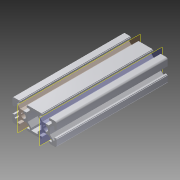
# Autodesk Inventor part: Dual Slotted Extrusion
Saved by Autodesk Inventor 2015 SP1 (Build 190203100, 203)
## iProperties
Created: 2015-03-03
Part Number: Dual Slotted Extrusion
Material: Aluminum 6061
Document SubType Name: Modeling
Designer: Andrew
Density: 2.7 g/cm^3
Appearance: Aluminum - Flat
Author: Andrew
Autodesk Inventor part; units mm, degrees
ref_plane "YZ Plane" through (0, 0, 0) normal (1, 0, 0) x (0, 1, 0)
ref_plane "XZ Plane" through (0, 0, 0) normal (0, 1, 0) x (-1, 0, 0)
ref_plane "XY Plane" through (0, 0, 0) normal (0, 0, 1) x (1, 0, 0)
sketch "Sketch1" plane through (0, 0, 0) normal (0, 1, 0) x (-1, 0, 0)
  line L0 (10, 10) -> (10, 3.6)
  line L1 (9.5, 3.1) -> (8, 3.1)
  line L2 (8, 3.1) -> (8, 5.63)
  line L3 (8, 5.63) -> (6.6907, 5.63)
  line L4 (6.6907, 5.63) -> (3.9, 2.8393)
  line L5 (2.8393, 3.9) -> (5.63, 6.6907)
  line L6 (5.63, 8) -> (5.63, 6.6907)
  line L7 (5.63, 8) -> (3.1, 8)
  line L8 (3.1, 8) -> (3.1, 9.5)
  line L9 (3.6, 10) -> (10, 10)
  line L10 (-2, 0) -> (12, 0) projected
  line L11 (0, -2) -> (0, 12) projected
  line L12 (3.9, 2.8393) -> (3.9, 0)
  line L13 (2.8393, 3.9) -> (0, 3.9)
  line L14 (0, 0) -> (10, 10) construction
  line L15 (10, 3.6) -> (9.5, 3.6)
  line L16 (9.5, 3.6) -> (9.5, 3.1)
  line L17 (3.6, 10) -> (3.6, 9.5)
  line L18 (3.6, 9.5) -> (3.1, 9.5)
  dimension "d0" = 45
  dimension "d1" = 5.63
  dimension "d2" = 10
  dimension "d3" = 3.1
  dimension "d5" = 6.1
  dimension "d6" = 1.5
  dimension "d7" = 2
  dimension "d11" = 3.6
  constraints: 34 end point, 12 perpendicular, 4 symmetric about line, 2 point on line, 2 vertical, 1 horizontal, 1 parallel, 1 other
  measures "d0" angle of L10 L14
  measures "d1" distance between parallel lines of L10 L3
  measures "d2" distance between parallel lines of L9 L10
  measures "d3" distance between parallel lines of L1 L10
  measures "d5" distance between parallel lines of L12 L0
  measures "d6" distance between parallel lines of L5 L4
  measures "d7" distance between parallel lines of L9 L7
  measures "d11" distance between parallel lines of L10 L15
extrude "Extrusion1" add sketch "Sketch1" along normal mid plane 100
fillet "Fillet1" radius 1.5 1 edges at (-10, 0, 10)
mirror "Mirror1" about plane through (0, 0, 3.9) normal (1, 0, 0)
mirror "Mirror2" about plane through (0, 0, 0) normal (0, 0, -1)
sketch "Sketch2" plane through (0, -50, 0) normal (0, -1, 0) x (1, 0, 0)
  circle A0 centre (0, 0) radius 2.225
  dimension "d12" = 4.45
  constraints: 1 centre point, 1 coincident
  measures "d12" diameter of A0
extrude "Extrusion2" cut sketch "Sketch2" against normal up to next
mirror "Mirror3" about plane through (10, 0, 3.6) normal (1, 0, 0)
sketch "Sketch3" plane through (0, -50, 0) normal (0, -1, 0) x (1, 0, 0)
  line L0 (9.5, -3.6) -> (10.5, -3.6) projected
  line L1 (9.5, -3.6) -> (9.5, -3.1) projected
  line L2 (9.5, -3.1) -> (8, -3.1) projected
  line L3 (8, -3.1) -> (8, -5.63) projected
  line L4 (8, -5.63) -> (6.6907, -5.63) projected
  line L5 (6.6907, -5.63) -> (3.9, -2.8393) projected
  line L6 (3.9, -2.8393) -> (3.9, 2.8393) projected
  line L7 (6.6907, 5.63) -> (3.9, 2.8393) projected
  line L8 (8, 5.63) -> (6.6907, 5.63) projected
  line L9 (8, 3.1) -> (8, 5.63) projected
  line L10 (9.5, 3.1) -> (8, 3.1) projected
  line L11 (9.5, 3.6) -> (9.5, 3.1) projected
  line L12 (10.5, 3.6) -> (9.5, 3.6) projected
  line L13 (10.5, 3.6) -> (10.5, 3.1) projected
  line L14 (10.5, 3.1) -> (12, 3.1) projected
  line L15 (12, 3.1) -> (12, 5.63) projected
  line L16 (12, 5.63) -> (13.3093, 5.63) projected
  line L17 (13.3093, 5.63) -> (16.1, 2.8393) projected
  line L18 (16.1, -2.8393) -> (16.1, 2.8393) projected
  line L19 (13.3093, -5.63) -> (16.1, -2.8393) projected
  line L20 (12, -5.63) -> (13.3093, -5.63) projected
  line L21 (12, -3.1) -> (12, -5.63) projected
  line L22 (10.5, -3.1) -> (12, -3.1) projected
  line L23 (10.5, -3.6) -> (10.5, -3.1) projected
  circle A0 centre (20, 0) radius 2.225 projected
  circle A1 centre (0, 0) radius 2.225 projected
  arc A2 (10, -8.5) -> (11.5, -10) centre (11.5, -8.5) ccw projected
  line L24 (16.4, -10) -> (11.5, -10) projected
  line L25 (16.4, -9.5) -> (16.4, -10) projected
  line L26 (16.9, -9.5) -> (16.4, -9.5) projected
  line L27 (16.9, -8) -> (16.9, -9.5) projected
  line L28 (14.37, -8) -> (16.9, -8) projected
  line L29 (14.37, -6.6907) -> (14.37, -8) projected
  line L30 (17.1607, -3.9) -> (14.37, -6.6907) projected
  line L31 (22.8393, -3.9) -> (17.1607, -3.9) projected
  line L32 (22.8393, -3.9) -> (25.63, -6.6907) projected
  line L33 (25.63, -6.6907) -> (25.63, -8) projected
  line L34 (25.63, -8) -> (23.1, -8) projected
  line L35 (23.1, -8) -> (23.1, -9.5) projected
  line L36 (23.1, -9.5) -> (23.6, -9.5) projected
  line L37 (23.6, -9.5) -> (23.6, -10) projected
  line L38 (23.6, -10) -> (28.5, -10) projected
  arc A3 (28.5, -10) -> (30, -8.5) centre (28.5, -8.5) ccw projected
  line L39 (30, -8.5) -> (30, -3.6) projected
  line L40 (30, -3.6) -> (29.5, -3.6) projected
  line L41 (29.5, -3.6) -> (29.5, -3.1) projected
  line L42 (29.5, -3.1) -> (28, -3.1) projected
  line L43 (28, -3.1) -> (28, -5.63) projected
  line L44 (28, -5.63) -> (26.6907, -5.63) projected
  line L45 (26.6907, -5.63) -> (23.9, -2.8393) projected
  line L46 (23.9, 2.8393) -> (23.9, -2.8393) projected
  line L47 (26.6907, 5.63) -> (23.9, 2.8393) projected
  line L48 (28, 5.63) -> (26.6907, 5.63) projected
  line L49 (28, 3.1) -> (28, 5.63) projected
  line L50 (29.5, 3.1) -> (28, 3.1) projected
  line L51 (29.5, 3.6) -> (29.5, 3.1) projected
  line L52 (30, 3.6) -> (29.5, 3.6) projected
  line L53 (30, 8.5) -> (30, 3.6) projected
  arc A4 (30, 8.5) -> (28.5, 10) centre (28.5, 8.5) ccw projected
  line L54 (23.6, 10) -> (28.5, 10) projected
  line L55 (23.6, 9.5) -> (23.6, 10) projected
  line L56 (23.1, 9.5) -> (23.6, 9.5) projected
  line L57 (23.1, 8) -> (23.1, 9.5) projected
  line L58 (25.63, 8) -> (23.1, 8) projected
  line L59 (25.63, 6.6907) -> (25.63, 8) projected
  line L60 (22.8393, 3.9) -> (25.63, 6.6907) projected
  line L61 (22.8393, 3.9) -> (17.1607, 3.9) projected
  line L62 (17.1607, 3.9) -> (14.37, 6.6907) projected
  line L63 (14.37, 6.6907) -> (14.37, 8) projected
  line L64 (14.37, 8) -> (16.9, 8) projected
  line L65 (16.9, 8) -> (16.9, 9.5) projected
  line L66 (16.9, 9.5) -> (16.4, 9.5) projected
  line L67 (16.4, 9.5) -> (16.4, 10) projected
  line L68 (16.4, 10) -> (11.5, 10) projected
  arc A5 (11.5, 10) -> (10, 8.5) centre (11.5, 8.5) ccw projected
  arc A6 (10, 8.5) -> (8.5, 10) centre (8.5, 8.5) ccw projected
  line L69 (3.6, 10) -> (8.5, 10) projected
  line L70 (3.6, 9.5) -> (3.6, 10) projected
  line L71 (3.1, 9.5) -> (3.6, 9.5) projected
  line L72 (3.1, 8) -> (3.1, 9.5) projected
  line L73 (5.63, 8) -> (3.1, 8) projected
  line L74 (5.63, 6.6907) -> (5.63, 8) projected
  line L75 (2.8393, 3.9) -> (5.63, 6.6907) projected
  line L76 (-2.8393, 3.9) -> (2.8393, 3.9) projected
  line L77 (-2.8393, 3.9) -> (-5.63, 6.6907) projected
  line L78 (-5.63, 6.6907) -> (-5.63, 8) projected
  line L79 (-5.63, 8) -> (-3.1, 8) projected
  line L80 (-3.1, 8) -> (-3.1, 9.5) projected
  line L81 (-3.1, 9.5) -> (-3.6, 9.5) projected
  line L82 (-3.6, 9.5) -> (-3.6, 10) projected
  line L83 (-3.6, 10) -> (-8.5, 10) projected
  arc A7 (-8.5, 10) -> (-10, 8.5) centre (-8.5, 8.5) ccw projected
  line L84 (-10, 8.5) -> (-10, 3.6) projected
  line L85 (-10, 3.6) -> (-9.5, 3.6) projected
  line L86 (-9.5, 3.6) -> (-9.5, 3.1) projected
  line L87 (-9.5, 3.1) -> (-8, 3.1) projected
  line L88 (-8, 3.1) -> (-8, 5.63) projected
  line L89 (-8, 5.63) -> (-6.6907, 5.63) projected
  line L90 (-6.6907, 5.63) -> (-3.9, 2.8393) projected
  line L91 (-3.9, 2.8393) -> (-3.9, -2.8393) projected
  line L92 (-6.6907, -5.63) -> (-3.9, -2.8393) projected
  line L93 (-8, -5.63) -> (-6.6907, -5.63) projected
  line L94 (-8, -3.1) -> (-8, -5.63) projected
  line L95 (-9.5, -3.1) -> (-8, -3.1) projected
  line L96 (-9.5, -3.6) -> (-9.5, -3.1) projected
  line L97 (-10, -3.6) -> (-9.5, -3.6) projected
  line L98 (-10, -8.5) -> (-10, -3.6) projected
  arc A8 (-10, -8.5) -> (-8.5, -10) centre (-8.5, -8.5) ccw projected
  line L99 (-3.6, -10) -> (-8.5, -10) projected
  line L100 (-3.6, -9.5) -> (-3.6, -10) projected
  line L101 (-3.1, -9.5) -> (-3.6, -9.5) projected
  line L102 (-3.1, -8) -> (-3.1, -9.5) projected
  line L103 (-5.63, -8) -> (-3.1, -8) projected
  line L104 (-5.63, -6.6907) -> (-5.63, -8) projected
  line L105 (-2.8393, -3.9) -> (-5.63, -6.6907) projected
  line L106 (-2.8393, -3.9) -> (2.8393, -3.9) projected
  line L107 (2.8393, -3.9) -> (5.63, -6.6907) projected
  line L108 (5.63, -6.6907) -> (5.63, -8) projected
  line L109 (5.63, -8) -> (3.1, -8) projected
  line L110 (3.1, -8) -> (3.1, -9.5) projected
  line L111 (3.1, -9.5) -> (3.6, -9.5) projected
  line L112 (3.6, -9.5) -> (3.6, -10) projected
  line L113 (3.6, -10) -> (8.5, -10) projected
  arc A9 (8.5, -10) -> (10, -8.5) centre (8.5, -8.5) ccw projected
  line L114 (8.5, 10) -> (11.5, 10)
  arc A10 (11.5, 10) -> (10, 8.5) centre (11.5, 8.5) ccw projected
  arc A11 (10, 8.5) -> (8.5, 10) centre (8.5, 8.5) ccw projected
  arc A12 (8.5, -10) -> (10, -8.5) centre (8.5, -8.5) ccw projected
  line L115 (6.6907, 5.63) -> (7.13, 6.0693)
  line L116 (7.13, 6.0693) -> (7.13, 8)
  line L117 (6.6907, 5.63) -> (8, 5.63) projected
  line L118 (7.13, 8) -> (12.87, 8)
  line L119 (12.87, 8) -> (12.87, 6.0693)
  line L120 (12.87, 6.0693) -> (13.3093, 5.63)
  line L121 (10.5, 3.6) -> (9.5, 3.6) construction
  line L122 (10, 3.6) -> (10, -3.6) construction
  line L123 (5.63, 8) -> (3.1, 8) construction
  line L124 (6.6907, 5.63) -> (3.9, 2.8393) construction
  line L125 (11.5, -10) -> (8.5, -10)
  line L126 (16.4, -10) -> (11.5, -10) projected
  dimension "d15" = 1.5
  constraints: 16 end point, 4 tangent, 3 collinear, 2 midpoint, 2 perpendicular, 1 horizontal, 1 symmetric about line, 1 vertical, 2 other
  measures "d15" distance between parallel lines of L74 L116
extrude "Extrusion3" cut sketch "Sketch3" against normal up to next contours L115 L116 L118 L119 L120 L16 L15 L14 L13 L12 L11 L10 L9 L8
extrude "Extrusion4" add sketch "Sketch3" against normal up to surface (100 mm away) contours A5 A6 L114
mirror "Mirror4" about plane through (0, 0, 0) normal (0, 0, 1) of "Extrusion3"
extrude "Extrusion5" add sketch "Sketch3" against normal up to surface (100 mm away) contours A2 L125 A9
ref_plane "Work Plane1" through (0, -50, 8) normal (1, 0, 0) x (0, 0, -1)
ref_plane "Work Plane2" through (20, -50, 8) normal (-1, 0, 0) x (0, 0, 1)
body "Solid1"
